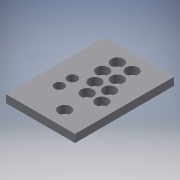
# Autodesk Inventor part: controlBoard
Saved by Autodesk Inventor 2017 (Build 210142000, 142)
## iProperties
Created: 2019-03-08
Part Number: controlBoard
Material: Generic
Document SubType Name: Modeling
Designer: Mitch
Density: 1 g/cm^3
Appearance: Default
Author: Mitch
Autodesk Inventor part; units mm, degrees
ref_plane "YZ Plane" through (0, 0, 0) normal (1, 0, 0) x (0, 1, 0)
ref_plane "XZ Plane" through (0, 0, 0) normal (0, 1, 0) x (-1, 0, 0)
ref_plane "XY Plane" through (0, 0, 0) normal (0, 0, 1) x (1, 0, 0)
sketch "Sketch1" plane through (0, 0, 0) normal (0, 1, 0) x (-1, 0, 0)
  line L0 (0, 0) -> (168.275, 0)
  line L1 (168.275, 0) -> (168.275, -241.3)
  line L2 (168.275, -241.3) -> (0, -241.3)
  line L3 (0, -241.3) -> (0, 0)
  dimension "d0" = 168.275
  dimension "d1" = 241.3
  constraints: 8 end point, 2 parallel, 1 horizontal, 1 perpendicular
  measures "d0" distance of L1.end L2.end
  measures "d1" distance of L0.end L1.end
extrude "Extrusion1" add sketch "Sketch1" along normal blind 19.05
sketch "Sketch2" plane through (0, 19.05, 0) normal (0, 1, 0) x (1, 0, 0)
  circle A0 centre (-63.5, 38.1) radius 14.986
  circle A1 centre (-71.501, 101.092) radius 14.986
  circle A2 centre (-85.471, 133.858) radius 14.986
  circle A3 centre (-99.441, 166.624) radius 14.986
  circle A4 centre (-99.441, 202.6158) radius 14.986
  circle A5 centre (-35.56, 101.092) radius 14.986
  circle A6 centre (-49.53, 133.858) radius 14.986
  circle A7 centre (-63.5, 166.624) radius 14.986
  circle A8 centre (-63.5, 202.6158) radius 14.986
  line L0 (0, 0) -> (-168.275, 0) projected
  circle A9 centre (-120.65, 82.55) radius 11.7475
  circle A10 centre (-120.65, 114.3) radius 11.7475
  line L1 (0, 0) -> (0, 241.3) projected
  dimension "d4" = 29.972
  dimension "d5" = 29.972
  dimension "d6" = 29.972
  dimension "d7" = 29.972
  dimension "d8" = 29.972
  dimension "d9" = 29.972
  dimension "d10" = 29.972
  dimension "d11" = 29.972
  dimension "d12" = 29.972
  dimension "d13" = 62.992
  dimension "d14" = 62.992
  dimension "d15" = 32.766
  dimension "d16" = 32.766
  dimension "d17" = 32.766
  dimension "d18" = 32.766
  dimension "d19" = 35.9918
  dimension "d20" = 35.9918
  dimension "d22" = 13.97
  dimension "d23" = 13.97
  dimension "d24" = 8.001
  dimension "d25" = 8.001
  dimension "d26" = 13.97
  dimension "d27" = 13.97
  dimension "d28" = 13.97
  dimension "d29" = 38.1
  dimension "d30" = 23.495
  dimension "d31" = 82.55
  dimension "d33" = 23.495
  dimension "d35" = 31.75
  dimension "d38" = 63.5
  dimension "d39" = 8.001
  dimension "d40" = 120.65
  dimension "d41" = 120.65
  constraints: 11 centre point
  measures "d4" diameter of A0
  measures "d5" diameter of A1
  measures "d6" diameter of A2
  measures "d7" diameter of A3
  measures "d8" diameter of A4
  measures "d9" diameter of A5
  measures "d10" diameter of A6
  measures "d11" diameter of A7
  measures "d12" diameter of A8
  measures "d13" vertical distance of A5.centre A0.centre
  measures "d14" vertical distance of A1.centre A0.centre
  measures "d15" vertical distance of A6.centre A5.centre
  measures "d16" vertical distance of A2.centre A1.centre
  measures "d17" vertical distance of A7.centre A6.centre
  measures "d18" vertical distance of A3.centre A2.centre
  measures "d19" distance of A8.centre A7.centre
  measures "d20" distance of A4.centre A3.centre
  measures "d22" horizontal distance of A4.centre A2.centre
  measures "d23" horizontal distance of A1.centre A2.centre
  measures "d24" horizontal distance of A8.centre A1.centre
  measures "d25" horizontal distance of A1.centre A7.centre
  measures "d26" horizontal distance of A6.centre A7.centre
  measures "d27" horizontal distance of A5.centre A6.centre
  measures "d28" horizontal distance of A2.centre A3.centre
  measures "d29" distance from line of L0 A0.centre
  measures "d30" diameter of A9
  measures "d31" distance from line of L0 A9.centre
  measures "d33" diameter of A10
  measures "d35" distance of A9.centre A10.centre
  measures "d38" distance from line of L1 A0.centre
  measures "d39" horizontal distance of A0.centre A1.centre
  measures "d40" distance from line of L1 A9.centre
  measures "d41" distance from line of L1 A10.centre
extrude "Extrusion2" cut sketch "Sketch2" against normal blind 25.4
body "Solid1"
